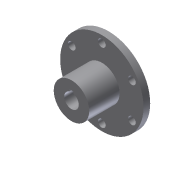
# Autodesk Inventor part: Hub 8mm key
Saved by Autodesk Inventor 2013 (Build 170138000, 138)
## iProperties
Created: 2012-06-03
Part Number: Hub 8mm key
Document SubType Name: Modeling
Designer: Nemo
Density: 1 g/cm^3
Material: Generic
Author: Nemo
Autodesk Inventor part; units mm, degrees
ref_plane "YZ Plane" through (0, 0, 0) normal (1, 0, 0) x (0, 1, 0)
ref_plane "XZ Plane" through (0, 0, 0) normal (0, 1, 0) x (-1, 0, 0)
ref_plane "XY Plane" through (0, 0, 0) normal (0, 0, 1) x (1, 0, 0)
sketch "Sketch1" plane through (0, 0, 0) normal (0, 0, 1) x (1, 0, 0)
  circle A0 centre (0, 0) radius 28.575
  dimension "d0" = 57.15
  constraints: 1 centre point, 1 coincident
  measures "d0" diameter of A0
extrude "Extrusion1" add sketch "Sketch1" along normal blind 4.572
sketch "Sketch2" plane through (0, 0, 4.572) normal (0, 0, 1) x (1, 0, 0)
  circle A0 centre (0, 0) radius 28.575 projected
  circle A1 centre (0, 0) radius 12.1666
  dimension "d3" = 24.3332
  constraints: 1 centre point, 1 coincident
  measures "d3" diameter of A1
extrude "Extrusion2" add sketch "Sketch2" along normal blind 20.828 contours A1
sketch "Sketch3" plane through (0, 0, 25.4) normal (0, 0, 1) x (1, 0, 0)
  circle A0 centre (0, 0) radius 12.1666 projected
  circle A1 centre (0, 0) radius 5
  line L0 (-1.25, 6.0912) -> (1.25, 6.0912)
  line L1 (1.25, 6.0912) -> (1.25, 3.5912)
  line L2 (1.25, 3.5912) -> (-1.25, 3.5912)
  line L3 (-1.25, 3.5912) -> (-1.25, 6.0912)
  point P0 (0, 6.0912)
  point P1 (-1.25, 4.8412)
  dimension "d6" = 10
  dimension "d7" = 2.5
  dimension "d8" = 2.5
  constraints: 8 end point, 2 midpoint, 2 parallel, 1 coincident, 1 horizontal, 1 perpendicular, 1 vertical alignment, 3 other
  measures "d7" distance of L1.end L2.end
  measures "d8" distance of L0.end L1.end
extrude "Extrusion3" cut sketch "Sketch3" against normal through all contours A1 L3 L2 L1 | L1 L2 L3 A1 | A1 L3 L0 L1
sketch "Sketch4" plane through (0, 0, 0) normal (0, 0, -1) x (-1, 0, 0)
  arc A0 (-1.25, 4.8412) -> (1.25, 4.8412) centre (0, 0) ccw projected
  circle A1 centre (0, 23.8125) radius 2.6162
  arc A2 (-1.25, 4.8412) -> (1.25, 4.8412) centre (0, 0) ccw projected
  line L0 (-1.25, 4.8412) -> (-1.25, 6.0912) projected
  line L1 (-1.25, 6.0912) -> (1.25, 6.0912) projected
  line L2 (1.25, 6.0912) -> (1.25, 4.8412) projected
  circle A3 centre (0, 0) radius 28.575 projected
  dimension "d11" = 5.2324
  dimension "d12" = 23.8125
  constraints: 1 centre point, 1 vertical alignment
  measures "d11" diameter of A1
  measures "d12" distance of A0.centre A1.centre
extrude "Extrusion4" cut sketch "Sketch4" against normal through all contours A1
pattern_circular "Circular Pattern1" count 6 over 360 about axis through (0, 0, 0) along (0, 0, 1) of "Extrusion4"
body "Solid1"
